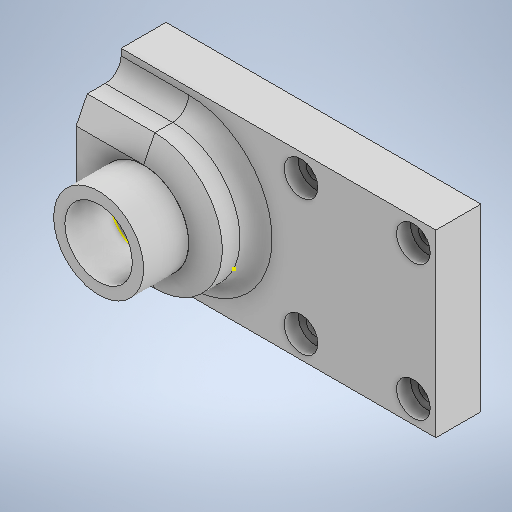
# Autodesk Inventor part: cad@49
Saved by Autodesk Inventor 2025.2 (Build 292293000, 293)
## iProperties
Created: 2025-04-08
Part Number: cad@49
Material: Generic
Document SubType Name: Modeling
Designer: spars
Density: 1 g/cm^3
Appearance: Default
Author: spars
Autodesk Inventor part; units mm, degrees
ref_plane "YZ Plane" through (0, 0, 0) normal (1, 0, 0) x (0, 1, 0)
ref_plane "XZ Plane" through (0, 0, 0) normal (0, 1, 0) x (-1, 0, 0)
ref_plane "XY Plane" through (0, 0, 0) normal (0, 0, 1) x (1, 0, 0)
sketch "Sketch1" plane through (0, 0, 0) normal (0, 0, 1) x (1, 0, 0)
  line L0 (-273.2587, 58.9048) -> (-103.4873, 58.9048) construction
  line L1 (-103.4873, 58.9048) -> (-103.4873, -61.7557) construction
  line L2 (-103.4873, -61.7557) -> (-273.2587, -61.7557) construction
  line L3 (-273.2587, -61.7557) -> (-273.2587, 58.9048) construction
  line L4 (-44.45, 25.4) -> (44.45, 25.4)
  line L5 (44.45, 25.4) -> (44.45, -25.4)
  line L6 (44.45, -25.4) -> (-44.45, -25.4)
  line L7 (-44.45, -25.4) -> (-44.45, 25.4)
  line L8 (-44.45, 25.4) -> (44.45, -25.4) construction
  line L9 (44.45, 25.4) -> (-44.45, -25.4) construction
  circle A0 centre (38.1, 19.05) radius 2.555
  circle A1 centre (6.35, 19.05) radius 2.555
  line L10 (0, 0) -> (70.2377, 0)
  circle A2 centre (38.1, -19.05) radius 2.555
  circle A3 centre (6.35, -19.05) radius 2.555
  dimension "d5" = 88.9
  dimension "d6" = 50.8
  dimension "d7" = 5.11
  dimension "d8" = 6.35
  dimension "d9" = 6.35
  dimension "d11" = 5.11
  constraints: 14 end point, 4 centre point, 2 horizontal, 2 midpoint, 2 parallel, 2 symmetric about line, 1 perpendicular, 4 other
  measures "d5" distance of L5.end L6.end
  measures "d6" distance of L4.end L5.end
  measures "d7" diameter of A0
  measures "d8" distance from line of L5 A0.centre
  measures "d9" distance from line of L4 A0.centre
  measures "d11" diameter of A1
extrude "Extrusion1" add sketch "Sketch1" along normal blind 12.7
sketch "Sketch2" plane through (0, 0, 12.7) normal (0, 0, 1) x (1, 0, 0)
  circle A0 centre (6.35, 19.05) radius 2.555 projected
  circle A1 centre (6.35, 19.05) radius 4.765
  circle A2 centre (38.1, 19.05) radius 2.555 projected
  circle A3 centre (38.1, 19.05) radius 4.765
  circle A4 centre (6.35, -19.05) radius 2.555 projected
  circle A5 centre (6.35, -19.05) radius 4.765
  circle A6 centre (38.1, -19.05) radius 2.555 projected
  circle A7 centre (38.1, -19.05) radius 4.765
  point P0 (0, 0)
  dimension "d19" = 9.53
  dimension "d20" = 9.53
  dimension "d21" = 9.53
  dimension "d22" = 9.53
  constraints: 4 centre point, 4 coincident
  measures "d19" diameter of A1
  measures "d20" diameter of A3
  measures "d21" diameter of A5
  measures "d22" diameter of A7
extrude "Extrusion2" cut sketch "Sketch2" against normal blind 4 contours A0 | A1 | A2 | A3 | A4 | A5 | A6 | A7
sketch "Sketch3" plane through (0, 0, 12.7) normal (0, 0, 1) x (1, 0, 0)
  line L0 (-44.45, 25.4) -> (-44.45, -25.4) projected
  line L1 (-44.45, -19.05) -> (-25.4, -19.05)
  line L2 (-44.45, 19.05) -> (-25.4, 19.05)
  arc A0 (-25.4, -19.05) -> (-25.4, 19.05) centre (-25.4, 0) ccw
  line L3 (-44.45, -19.05) -> (-44.45, 19.05)
  point P0 (0, 0)
  dimension "d25" = 19.05
  dimension "d26" = 19.05
  dimension "d29" = 19.05
  constraints: 6 end point, 2 point on circle, 2 point on line, 1 centre point, 1 collinear, 1 horizontal, 1 perpendicular
  measures "d25" distance of L1.start L1.end
  measures "d26" distance of L2.start L2.end
  measures "d29" radius of A0
extrude "Extrusion3" add sketch "Sketch3" along normal blind 12.7
fillet "Face Fillet1" radius 4.5 1 edges at (-34.925, -19.05, 12.7)
sketch "Sketch4" plane through (0, 0, 25.4) normal (0, 0, 1) x (1, 0, 0)
  arc A0 (-25.4, -19.05) -> (-25.4, 19.05) centre (-25.4, 0) ccw projected
  line L0 (-44.45, 19.05) -> (-44.45, -19.05) projected
  line L1 (-44.45, -12.7) -> (-44.45, 12.7)
  point P0 (0, 0)
  constraints: 2 end point, 2 point on line, 1 collinear
extrude "Extrusion4" [suppressed]
sketch "Sketch5" plane through (0, 0, 25.4) normal (0, 0, 1) x (1, 0, 0)
  arc A0 (-25.4, -19.05) -> (-25.4, 19.05) centre (-25.4, 0) ccw projected
  circle A1 centre (-25.4, 0) radius 12.7
  circle A2 centre (-25.4, 0) radius 9.525
  point P0 (0, 0)
  dimension "d38" = 25.4
  dimension "d39" = 19.05
  constraints: 2 centre point, 2 coincident
  measures "d38" diameter of A1
  measures "d39" diameter of A2
extrude "Extrusion5" add sketch "Sketch5" along normal blind 12.7
chamfer "Chamfer1" distance 6.3 angle 26.6 3 edges at (-34.925, -19.05, 25.4) (-6.35, 0, 25.4) (-34.925, 19.05, 25.4) measured on face at (-42.3333, 0, 25.4)
sketch "Sketch6" plane through (-25.4, 0, 25.4) normal (0, 0, 1) x (1, 0, 0)
  circle A0 centre (0, 0) radius 9.525 projected
  circle A1 centre (0, 0) radius 9.525
  point P0 (25.4, 0)
  constraints: 1 centre point, 1 coincident
body "Solid1"
